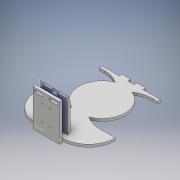
# Autodesk Inventor part: new_base
Saved by Autodesk Inventor 2018 (Build 220112000, 112)
## iProperties
Created: 2018-05-04
Part Number: new_base
Material: Generic
Document SubType Name: Modeling
Designer: rfabre
Density: 1 g/cm^3
Appearance: Default
Author: rfabre
Autodesk Inventor part; units mm, degrees
ref_plane "YZ Plane" through (0, 0, 0) normal (1, 0, 0) x (0, 1, 0)
ref_plane "XZ Plane" through (0, 0, 0) normal (0, 1, 0) x (-1, 0, 0)
ref_plane "XY Plane" through (0, 0, 0) normal (0, 0, 1) x (1, 0, 0)
sketch "Sketch1" plane through (0, 0, 0) normal (0, 1, 0) x (-1, 0, 0)
  line L0 (0, 0) -> (50, 0)
  line L1 (50, 0) -> (50, -70)
  line L2 (50, -70) -> (0, -70)
  line L3 (0, -70) -> (0, 0)
  line L4 (25, 0) -> (25, -70) construction
  line L5 (31, -70) -> (19, -70) construction
  line L6 (19, -70) -> (19, 0) construction
  line L7 (19, 0) -> (31, 0) construction
  line L8 (31, 0) -> (31, -70) construction
  line L9 (31, -70) -> (19, -70) construction
  line L10 (19, -70) -> (19, -41.2) construction
  line L11 (19, -41.2) -> (31, -41.2) construction
  line L12 (31, -41.2) -> (31, -70) construction
  line L13 (31, 0) -> (19, 0) construction
  line L14 (19, 0) -> (19, -28.8) construction
  line L15 (19, -28.8) -> (31, -28.8) construction
  line L16 (31, -28.8) -> (31, 0) construction
  line L17 (46.6733, -3.3267) -> (3.3267, -3.3267) construction
  line L18 (3.3267, -3.3267) -> (3.3267, -66.6733) construction
  line L19 (3.3267, -66.6733) -> (46.6733, -66.6733) construction
  line L20 (46.6733, -66.6733) -> (46.6733, -3.3267) construction
  line L21 (46.6733, -3.3267) -> (31.2367, -3.3267)
  line L22 (31.2367, -3.3267) -> (31.2367, -7.9167)
  line L23 (31.2367, -7.9167) -> (46.6733, -7.9167)
  line L24 (46.6733, -7.9167) -> (46.6733, -3.3267)
  line L25 (46.6733, -66.6733) -> (31.2367, -66.6733)
  line L26 (31.2367, -66.6733) -> (31.2367, -62.0833)
  line L27 (31.2367, -62.0833) -> (46.6733, -62.0833)
  line L28 (46.6733, -62.0833) -> (46.6733, -66.6733)
  line L29 (3.3267, -66.6733) -> (18.7633, -66.6733)
  line L30 (18.7633, -66.6733) -> (18.7633, -62.0833)
  line L31 (18.7633, -62.0833) -> (3.3267, -62.0833)
  line L32 (3.3267, -62.0833) -> (3.3267, -66.6733)
  line L33 (3.3267, -3.3267) -> (18.7633, -3.3267)
  line L34 (18.7633, -3.3267) -> (18.7633, -7.9167)
  line L35 (18.7633, -7.9167) -> (3.3267, -7.9167)
  line L36 (3.3267, -7.9167) -> (3.3267, -3.3267)
  circle A0 centre (17.7, -20) radius 1.3
  circle A1 centre (32.3, -20) radius 1.3
  circle A2 centre (32.3, -50) radius 1.3
  circle A3 centre (17.7, -50) radius 1.3
  dimension "d0" = 70
  dimension "d1" = 50
  dimension "d6" = 12
  dimension "d8" = 28.8
  dimension "d10" = 28.8
  dimension "d16" = 3.3267
  dimension "d17" = 3.3267
  dimension "d18" = 3.3267
  dimension "d19" = 3.3267
  dimension "d20" = 4.59
  dimension "d21" = 15.4367
  dimension "visse_dist" = 20
  dimension "d26" = 2.6
  dimension "d27" = 20
  dimension "d28" = 20
  dimension "d29" = 20
  constraints: 74 end point, 18 parallel, 9 horizontal, 9 perpendicular, 8 point on line, 4 centre point, 4 tangent, 3 equal radius, 3 midpoint, 2 equal length
  measures "d0" distance of L2.end L0.start
  measures "d1" distance of L0.start L0.end
  measures "d6" distance between parallel lines of L6 L8
  measures "d8" distance from line of L2 L11.end
  measures "d10" distance of L13.end L14.end
  measures "d16" distance between parallel lines of L0 L17
  measures "d17" distance between parallel lines of L1 L20
  measures "d18" distance between parallel lines of L2 L19
  measures "d19" distance between parallel lines of L3 L18
  measures "d20" distance of L21.end L22.end
  measures "d21" distance of L22.end L23.end
  measures "visse_dist" distance from line of L0 A0.centre
  measures "d26" diameter of A0
  measures "d27" distance from line of L0 A1.centre
  measures "d28" distance from line of L2 A2.centre
  measures "d29" distance from line of L2 A3.centre
extrude "Extrusion2" add sketch "Sketch1" along normal blind 4.99
ref_plane "Work Plane1" through (0, 14.99, 0) normal (0, 1, 0) x (1, 0, 0)
ref_plane "Work Plane2" through (-31.2367, 0, -62.0833) normal (0, 0, -1) x (-1, 0, 0)
sketch "Sketch3" plane through (-31.2367, 0, -62.0833) normal (0, 0, -1) x (-1, 0, 0)
  line L0 (0, 0) -> (16.2367, 0)
  line L1 (16.2367, 0) -> (16.2367, 5.39)
  line L2 (16.2367, 5.39) -> (19, 5.39)
  line L3 (0, 0) -> (0, 5.39)
  line L4 (0, 5.39) -> (-12, 5.39) construction
  line L5 (-12, 5.39) -> (-12, 0)
  line L6 (-12, 0) -> (-28.2367, 0)
  line L7 (-28.2367, 0) -> (-28.2367, 5.39)
  line L8 (-28.2367, 5.39) -> (-31, 5.39)
  arc A0 (19, 5.39) -> (69, 55.39) centre (19, 55.39) ccw
  line L9 (19, 55.39) -> (69, 55.39) construction
  arc A1 (-81, 55.39) -> (-31, 5.39) centre (-31, 55.39) ccw
  line L10 (-81, 55.39) -> (-31, 55.39) construction
  line L11 (-81, 55.39) -> (-51, 55.39)
  line L12 (69, 55.39) -> (39, 55.39)
  line L13 (-61, 155.39) -> (-51, 155.39)
  arc A2 (39, 155.39) -> (9.8333, 146.0016) centre (39, 105.39) ccw
  arc A3 (-51, 55.39) -> (-21.8333, 64.7784) centre (-51, 105.39) ccw
  line L14 (-51, 105.39) -> (39, 105.39) construction
  arc A4 (-21.8333, 146.0016) -> (-21.8333, 64.7784) centre (-6, 105.39) ccw
  arc A5 (-21.8333, 146.0016) -> (-51, 155.39) centre (-51, 105.39) ccw
  arc A6 (9.8333, 146.0016) -> (9.8333, 64.7784) centre (39, 105.39) ccw construction
  arc A7 (9.8333, 64.7784) -> (39, 55.39) centre (39, 105.39) ccw
  arc A8 (-21.8333, 64.7784) -> (-21.8333, 146.0016) centre (-51, 105.39) ccw construction
  arc A9 (9.8333, 146.0016) -> (-21.8333, 146.0016) centre (-6, 105.39) ccw construction
  arc A10 (9.8333, 64.7784) -> (9.8333, 146.0016) centre (-6, 105.39) ccw
  arc A11 (-21.8333, 64.7784) -> (9.8333, 64.7784) centre (-6, 105.39) ccw construction
  line L15 (-51, 155.39) -> (39, 155.39) construction
  line L16 (39, 155.39) -> (49, 155.39)
  line L17 (-61, 155.39) -> (-61, 160.39)
  line L18 (49, 160.39) -> (49, 155.39)
  line L19 (49, 160.39) -> (16.2367, 160.39)
  line L20 (16.2367, 160.39) -> (16.2367, 165.78)
  line L21 (16.2367, 165.78) -> (0, 165.78)
  line L22 (0, 165.78) -> (0, 160.39)
  line L23 (0, 160.39) -> (-12, 160.39)
  line L24 (-12, 160.39) -> (-12, 165.78)
  line L25 (-12, 165.78) -> (-28.2367, 165.78)
  line L26 (-28.2367, 165.78) -> (-28.2367, 160.39)
  line L27 (-28.2367, 160.39) -> (-61, 160.39)
  line L28 (-27.4367, 14.99) -> (-12, 14.99)
  line L29 (-12, 14.99) -> (-12, 19.58)
  line L30 (-12, 19.58) -> (-27.4367, 19.58)
  line L31 (-27.4367, 19.58) -> (-27.4367, 14.99)
  line L32 (0, 14.99) -> (15.4367, 14.99)
  line L33 (15.4367, 14.99) -> (15.4367, 19.58)
  line L34 (15.4367, 19.58) -> (0, 19.58)
  line L35 (0, 19.58) -> (0, 14.99)
  line L36 (-125.4975, 14.99) -> (113.4975, 14.99) construction
  line L37 (-12, 14.99) -> (0, 14.99) construction
  line L38 (-12, 17.285) -> (0, 17.285) construction
  line L39 (-12, 5.39) -> (-12, 14.99)
  line L40 (-12, 14.99) -> (0, 14.99)
  line L41 (0, 14.99) -> (0, 5.39)
  point P0 (-31.2367, 0)
  point P1 (-6, 5.39)
  point P2 (-6, 83.5955)
  point P3 (-28.2367, 14.99)
  point P4 (16.2367, 14.99)
  point P5 (-6, 14.99)
  point P6 (-6, 17.285)
  point P7 (18.7633, 4.99)
  dimension "d34" = 16.2367
  dimension "d35" = 5.39
  dimension "d36" = 12
  dimension "d37" = 50
  dimension "body_extra_r" = 50
  dimension "body_angle" = 90
  dimension "d42" = 50
  dimension "d43" = 90
  dimension "d45" = 150
  dimension "extra_flat" = 30
  dimension "d48" = 21.7945
  dimension "d49" = 87.178
  dimension "d50" = 10
  dimension "d51" = 5
  dimension "d65" = 4.59
  dimension "d66" = 15.4367
  dimension "d67" = 3.3267
  dimension "d68" = 9.6
  constraints: 82 end point, 32 point on circle, 16 perpendicular, 15 point on line, 14 tangent, 12 centre point, 11 equal length, 8 horizontal, 6 midpoint, 5 parallel, 3 collinear, 3 vertical, 2 vertical alignment, 1 coincident
  measures "d34" distance of L0.start L0.end
  measures "d35" distance of L0.end L1.end
  measures "d36" distance of L3.end L4.end
  measures "d37" distance of L2.end L8.end
  measures "body_extra_r" radius of A0
  measures "body_angle" angle of L9 L1
  measures "d42" radius of A1
  measures "d43" angle of L7 L10
  measures "d45" distance between parallel lines of L8 L13
  measures "extra_flat" distance of L10.start L11.end
  measures "d48" distance of point (-6, 83.596) A4.centre
  measures "d49" diameter of A4
  measures "d50" distance of L13.start L13.end
  measures "d51" distance of L18.start L16.end
  measures "d65" distance of L28.end L29.end
  measures "d66" distance of L29.end L30.end
  measures "d67" distance from line of L33 point (18.763, 4.99)
  measures "d68" distance of L40.end L3.end
sketch "Sketch4" plane through (-31.2367, 0, -62.0833) normal (0, 0, -1) x (-1, 0, 0)
  point P0 (-31.2367, 0)
sketch "Sketch5" plane through (0, 14.99, 0) normal (0, 1, 0) x (1, 0, 0)
  line L0 (0, 0) -> (0, 70) construction
  line L1 (0, 62.0833) -> (0, 35) construction
  line L2 (-50, 0) -> (0, 0) construction
  line L3 (-50, 70) -> (-50, 0) construction
  line L4 (-50, 7.9167) -> (-50, 35)
  line L5 (-46.6733, 7.9167) -> (-31.2367, 7.9167) construction
  line L6 (-18.7633, 7.9167) -> (-3.3267, 7.9167) construction
  line L7 (0, 70) -> (-50, 70) construction
  line L8 (-50, 7.9167) -> (0, 7.9167) construction
  line L9 (-3.3267, 7.9167) -> (-18.7633, 7.9167) construction
  line L10 (-50, 7.9167) -> (-47.0733, 7.9167)
  line L11 (-47.0733, 2.9267) -> (-30.8367, 2.9267)
  line L12 (-30.8367, 2.9267) -> (-30.8367, 7.9167)
  line L13 (-19.1633, 7.9167) -> (-19.1633, 2.9267)
  line L14 (-19.1633, 2.9267) -> (-2.9267, 2.9267)
  line L15 (-47.0733, 2.9267) -> (-47.0733, 7.9167)
  line L16 (-30.8367, 7.9167) -> (-19.1633, 7.9167)
  line L17 (-46.6733, 3.3267) -> (-46.6733, 7.9167) construction
  line L18 (-31.2367, 7.9167) -> (-31.2367, 3.3267) construction
  line L19 (-18.7633, 3.3267) -> (-18.7633, 7.9167) construction
  line L20 (-3.3267, 7.9167) -> (-3.3267, 3.3267) construction
  line L21 (-46.6733, 5.6217) -> (-31.2367, 5.6217) construction
  line L22 (-18.7633, 7.9167) -> (-18.7633, 3.3267) construction
  line L23 (-18.7633, 5.6217) -> (-3.3267, 5.6217) construction
  line L24 (-2.9267, 2.9267) -> (-2.9267, 7.9167)
  line L25 (0, 7.9167) -> (-2.9267, 7.9167)
  line L26 (-50, 35) -> (0, 35) construction
  line L27 (-50, 35) -> (-50, 62.0833) construction
  line L28 (0, 35) -> (0, 7.9167)
  line L29 (-50, 35) -> (-50, 57.515) construction
  line L30 (-50, 35) -> (-50, 35)
  line L31 (-3.3267, 62.0833) -> (-18.7633, 62.0833) construction
  line L32 (-11.045, 62.0833) -> (-11.045, 7.9167) construction
  line L33 (-50, 35) -> (-50, 62.0833)
  line L34 (-50, 62.0833) -> (-47.0733, 62.0833)
  line L35 (-47.0733, 62.0833) -> (-47.0733, 67.0733)
  line L36 (-47.0733, 67.0733) -> (-30.8367, 67.0733)
  line L37 (-30.8367, 67.0733) -> (-30.8367, 62.0833)
  line L38 (-30.8367, 62.0833) -> (-19.1633, 62.0833)
  line L39 (-19.1633, 62.0833) -> (-19.1633, 67.0733)
  line L40 (-19.1633, 67.0733) -> (-2.9267, 67.0733)
  line L41 (-2.9267, 67.0733) -> (-2.9267, 62.0833)
  line L42 (-2.9267, 62.0833) -> (0, 62.0833)
  line L43 (0, 62.0833) -> (0, 35)
  circle A0 centre (-32.3, 20) radius 1.3 projected
  circle A1 centre (-32.3, 50) radius 1.3 projected
  circle A2 centre (-17.7, 50) radius 1.3 projected
  circle A3 centre (-17.7, 20) radius 1.3 projected
  line L44 (-32, 32.7267) -> (-18, 32.7267)
  line L45 (-18, 32.7267) -> (-18, 24.3267)
  line L46 (-18, 24.3267) -> (-32, 24.3267)
  line L47 (-32, 24.3267) -> (-32, 32.7267)
  line L48 (-50, 31.7267) -> (0, 31.7267) construction
  line L49 (-32, 37.2733) -> (-18, 37.2733)
  line L50 (-18, 37.2733) -> (-18, 45.6733)
  line L51 (-18, 45.6733) -> (-32, 45.6733)
  line L52 (-32, 45.6733) -> (-32, 37.2733)
  point P0 (-25, 7.9167)
  point P1 (-38.955, 5.6217)
  point P2 (-38.955, 2.9267)
  point P3 (-11.045, 5.6217)
  point P4 (-11.045, 2.9267)
  point P5 (-11.045, 35)
  point P6 (-25, 24.3267)
  point P7 (-25, 7.9167)
  point P8 (-32, 28.5267)
  dimension "d55" = 4.99
  dimension "d56" = 16.2367
  dimension "d57" = 14
  dimension "d58" = 8.4
  dimension "d61" = 28.8
  dimension "motor_margin" = 1
  constraints: 80 end point, 22 point on line, 17 midpoint, 10 perpendicular, 7 equal length, 5 collinear, 4 horizontal, 4 symmetric about line, 3 parallel, 3 vertical alignment, 2 vertical
  measures "d55" distance of L13.start L13.end
  measures "d56" distance of L11.start L11.end
  measures "d57" distance of L45.end L46.end
  measures "d58" distance of L44.end L45.end
  measures "d61" distance between parallel lines of L11 L48
  measures "motor_margin" distance between parallel lines of L44 L48
extrude "Extrusion4" add sketch "Sketch5" along normal blind 4.99 separate body
extrude "Extrusion5" add sketch "Sketch3" along normal blind 4.99 bodies 1
equation "\"d0\" = base_L"
equation "\"d1\" = base_l"
equation "\"d6\" = motor_width"
equation "\"d8\" = extrud1 + extrud3"
equation "\"d10\" = d8"
equation "\"d16\" = extra_wood"
equation "\"d17\" = d16"
equation "\"d18\" = d16"
equation "\"d19\" = d17"
equation "\"d20\" = fente_l"
equation "\"d21\" = fente_L"
equation "\"d26\" = vis_moteur_d"
equation "\"d27\" = visse_dist"
equation "\"d28\" = visse_dist"
equation "\"d29\" = visse_dist"
equation "\"d30\" = thick"
equation "\"d34\" = male_L"
equation "\"d35\" = male_l"
equation "\"d36\" = motor_width"
equation "\"d37\" = base_l"
equation "\"d42\" = body_extra_r"
equation "\"d43\" = body_angle"
equation "\"base_L\" = 70"
equation "\"base_l\" = 50"
equation "\"motor_width\" = 12"
equation "\"extrud1\" = 22.4"
equation "\"extrud3\" = 6.4"
equation "\"extra_wood\" = 3.326667"
equation "\"fente_l\" = 4.59"
equation "\"fente_L\" = 15.436667"
equation "\"vis_moteur_d\" = 2.6"
equation "\"thick\" = 4.99"
equation "\"male_L\" = 16.236667"
equation "\"male_l\" = 5.39"
body "Solid3"
body "Solid5"
